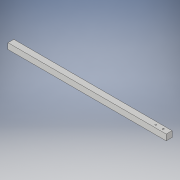
# Autodesk Inventor part: jewlArmBeam
Saved by Autodesk Inventor 2017 (Build 210142000, 142)
## iProperties
Created: 2017-10-14
Part Number: jewlArmBeam
Material: Generic
Document SubType Name: Modeling
Designer: User
Density: 1 g/cm^3
Appearance: Default
Author: User
Autodesk Inventor part; units mm, degrees
ref_plane "YZ Plane" through (0, 0, 0) normal (1, 0, 0) x (0, 1, 0)
ref_plane "XZ Plane" through (0, 0, 0) normal (0, 1, 0) x (-1, 0, 0)
ref_plane "Work Plane1" through (0, 0, 3.175) normal (0, 0, 1) x (1, 0, 0)
sketch "Sketch1" plane through (0, 0, 3.175) normal (0, 0, 1) x (1, 0, 0)
  line L0 (0, 0) -> (342.9, 0)
  line L1 (342.9, 0) -> (342.9, 12.7)
  line L2 (342.9, 12.7) -> (0, 12.7)
  line L3 (0, 12.7) -> (0, 0)
  dimension "d1" = 342.9
  dimension "d2" = 12.7
  constraints: 8 end point, 2 parallel, 1 horizontal, 1 perpendicular
  measures "d1" distance of L2.end L1.end
  measures "d2" distance of L1.end L0.end
extrude "Extrusion1" add sketch "Sketch1" along normal blind 12.7
sketch "Sketch2" plane through (0, 12.7, 3.175) normal (0, 1, 0) x (1, 0, 0)
  circle A0 centre (330.2, -6.35) radius 1.5875
  line L0 (0, 0) -> (342.9, 0) projected
  line L1 (342.9, 0) -> (342.9, -12.7) projected
  circle A1 centre (314.198, -6.35) radius 1.5875
  point P0 (0, 3.175)
  dimension "d5" = 6.35
  dimension "d6" = 3.175
  dimension "d7" = 12.7
  dimension "d8" = 3.175
  dimension "d9" = 6.35
  dimension "d10" = 16.002
  constraints: 2 centre point
  measures "d5" distance from line of L0 A0.centre
  measures "d6" diameter of A0
  measures "d7" distance from line of L1 A0.centre
  measures "d8" diameter of A1
  measures "d9" distance from line of L0 A1.centre
  measures "d10" distance of A0.centre A1.centre
extrude "Extrusion2" add sketch "Sketch2" along normal blind 0.254
body "Solid1"
